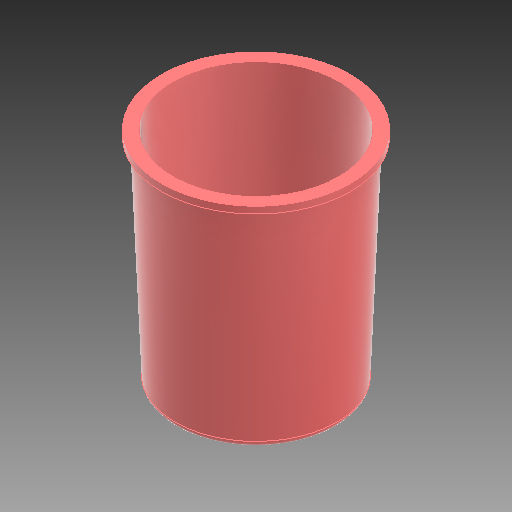
# Autodesk Inventor part: Стакан_В2
Saved by Autodesk Inventor 2022 (Build 260153000, 153)
## iProperties
Created: 2025-01-17
Part Number: Стакан_В2
Material: Типовые
Document SubType Name: Modeling
Designer: Ivan
Density: 1 g/cm^3
Appearance: Гладкий — красный
Mass: 22.4408 g
Surface Area: 227.827 cm^2
Volume: 22.4408 cm^3
Author: Ivan
Title: Стакан_В2
Autodesk Inventor part; units mm, degrees
ref_plane "YZ Plane" through (0, 0, 0) normal (1, 0, 0) x (0, 1, 0)
ref_plane "XZ Plane" through (0, 0, 0) normal (0, 1, 0) x (-1, 0, 0)
ref_plane "XY Plane" through (0, 0, 0) normal (0, 0, 1) x (1, 0, 0)
sketch "Эскиз1" plane through (0, 0, 0) normal (0, 0, 1) x (1, 0, 0)
  line L0 (0, 0) -> (0, 57.7087)
  line L1 (0, 0) -> (87.3611, 0) construction
  line L2 (21.4984, 0) -> (24.079, 64)
  line L3 (24.079, 64) -> (27.5, 64)
  line L4 (27.5, 64) -> (27.5, 62)
  line L5 (27.5, 62) -> (26, 62)
  line L6 (26, 62) -> (23.5, 0)
  line L7 (21.4984, 0) -> (23.5, 0)
  line L8 (23.5, 0) -> (0, 0)
  line L9 (0, 0) -> (0, 2)
  line L10 (0, 2) -> (21.579, 2)
  dimension "d0" = 47
  dimension "d1" = 52
  dimension "d2" = 55
  dimension "d3" = 62
  dimension "d4" = 2
  dimension "d5" = 2
  dimension "d8" = 2
  constraints: 22 end point, 4 point on line, 3 perpendicular, 2 collinear, 2 horizontal, 1 parallel, 1 vertical
  measures "d0" diameter of L6.end L0
  measures "d1" diameter of L5.end L0
  measures "d2" diameter of L4 L0
  measures "d3" distance between parallel lines of L1 L5
  measures "d4" distance of L3.end L4.end
  measures "d5" distance between parallel lines of L6 L2
  measures "d8" distance between parallel lines of L1 L10
revolve "Вращение1" add sketch "Эскиз1" angle 360 about axis through (0, 0, 0) along (0, 1, 0)
fillet "Сопряжение1" radius 2 1 edges at (-23.5, 0, 0)
equation "\"d8\" = d4"
